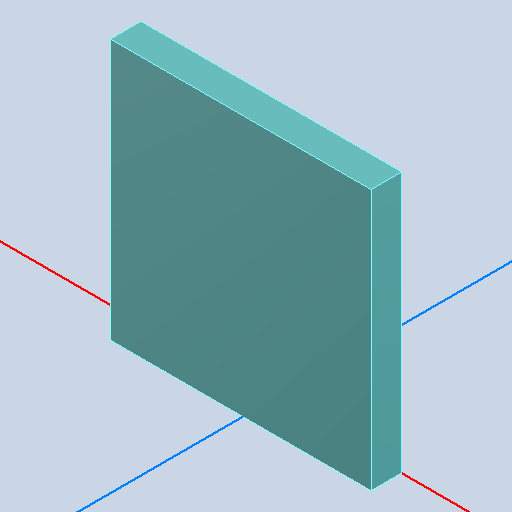
# Autodesk Inventor part: 153CLV-0810
Saved by Autodesk Inventor 2022 (Build 260153000, 153)
## iProperties
Created: 2022-12-24
Part Number: 153CLV-0810
Material: Типовые
Document SubType Name: Modeling
Designer: Ivan Petrov
Density: 1 g/cm^3
Appearance: 153CLV-0810, 153CLV-0810
Author: Ivan Petrov
Autodesk Inventor part; units mm, degrees
ref_plane "YZ Plane" through (0, 0, 0) normal (1, 0, 0) x (0, 1, 0)
ref_plane "XZ Plane" through (0, 0, 0) normal (0, 1, 0) x (-1, 0, 0)
ref_plane "XY Plane" through (0, 0, 0) normal (0, 0, 1) x (1, 0, 0)
sketch "153CLV-0810, 153CLV-0810_10" plane through (0, 0, 0) normal (0, 0, 1) x (1, 0, 0)
  line L0 (-4.3016, 4.2) -> (4.2, 4.2)
  line L1 (4.2, 4.2) -> (4.2, -4.3016)
  line L2 (4.2, -4.3016) -> (-4.3016, -4.3016)
  line L3 (-4.3016, -4.3016) -> (-4.3016, 4.2)
  constraints: 8 end point
extrude "Выдавливание1" add sketch "153CLV-0810, 153CLV-0810_10" along normal blind 1
